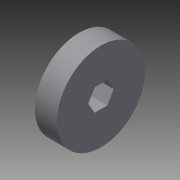
# Autodesk Inventor part: back roller hub
Saved by Autodesk Inventor 2015 SP1 (Build 190203100, 203)
## iProperties
Created: 2015-01-25
Part Number: back roller hub
Material: Generic
Document SubType Name: Modeling
Designer: Admin
Density: 1 g/cm^3
Appearance: Default
Author: Admin
Autodesk Inventor part; units mm, degrees
ref_plane "YZ Plane" through (0, 0, 0) normal (1, 0, 0) x (0, 1, 0)
ref_plane "XZ Plane" through (0, 0, 0) normal (0, 1, 0) x (-1, 0, 0)
ref_plane "XY Plane" through (0, 0, 0) normal (0, 0, 1) x (1, 0, 0)
sketch "Sketch1" plane through (0, 0, 0) normal (1, 0, 0) x (0, 1, 0)
  circle A0 centre (0, 0) radius 25.4
  dimension "d0" = 50.8
  constraints: 1 centre point, 1 coincident
  measures "d0" diameter of A0
extrude "Extrusion1" add sketch "Sketch1" along normal blind 12.7
sketch "Sketch2" plane through (12.7, 0, 0) normal (1, 0, 0) x (0, 0, -1)
  circle A0 centre (0, 0) radius 25.4 projected
  line L0 (-3.6662, 6.35) -> (3.6662, 6.35)
  line L1 (3.6662, 6.35) -> (7.3323, 0)
  line L2 (7.3323, 0) -> (3.6662, -6.35)
  line L3 (3.6662, -6.35) -> (-3.6662, -6.35)
  line L4 (-3.6662, -6.35) -> (-7.3323, 0)
  line L5 (-7.3323, 0) -> (-3.6662, 6.35)
  dimension "d3" = 12.7
  dimension "d4" = 12.7
  dimension "d5" = 12.7
  dimension "d6" = 6.35
  dimension "d7" = 6.35
  dimension "d8" = 6.35
  dimension "d9" = 120
  dimension "d10" = 120
  constraints: 12 end point, 3 parallel, 1 horizontal
  measures "d3" distance between parallel lines of L3 L0
  measures "d4" distance between parallel lines of L4 L1
  measures "d5" distance between parallel lines of L2 L5
  measures "d6" distance from line of A0.centre L0
  measures "d7" distance from line of A0.centre L1
  measures "d8" distance from line of A0.centre L5
  measures "d9" angle of L0 L5
  measures "d10" angle of L1 L0
extrude "Extrusion2" cut sketch "Sketch2" against normal blind 12.7 contours L0 L1 L2 L3 L4 L5
body "Solid1"
